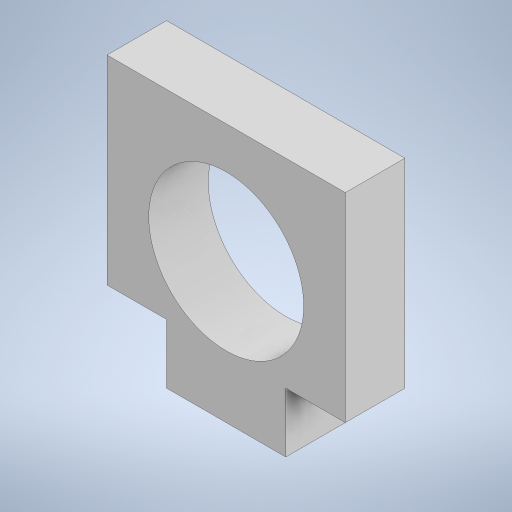
# Autodesk Inventor part: rod holder
Saved by Autodesk Inventor 2023 (Build 270158000, 158)
## iProperties
Created: 2023-11-14
Part Number: rod holder
Material: Generic
Document SubType Name: Modeling
Designer: Nate
Density: 1 g/cm^3
Appearance: Default
Author: Nate
Autodesk Inventor part; units mm, degrees
ref_plane "YZ Plane" through (0, 0, 0) normal (1, 0, 0) x (0, 1, 0)
ref_plane "XZ Plane" through (0, 0, 0) normal (0, 1, 0) x (-1, 0, 0)
ref_plane "XY Plane" through (0, 0, 0) normal (0, 0, 1) x (1, 0, 0)
sketch "Sketch1" plane through (0, 0, 0) normal (0, 0, 1) x (1, 0, 0)
  circle A0 centre (0, 0) radius 4.1275
  line L0 (-6.35, 6.35) -> (6.35, 6.35)
  line L1 (6.35, 6.35) -> (6.35, -4.2672)
  line L2 (6.35, -4.2672) -> (-6.35, -4.2672)
  line L3 (-6.35, -4.2672) -> (-6.35, 6.35)
  line L4 (-3.175, -4.2672) -> (3.175, -4.2672)
  line L5 (3.175, -4.2672) -> (3.175, -7.4422)
  line L6 (3.175, -7.4422) -> (-3.175, -7.4422)
  line L7 (-3.175, -7.4422) -> (-3.175, -4.2672)
  dimension "d0" = 8.255
  dimension "d1" = 4.2672
  dimension "d2" = 6.35
  dimension "d3" = 6.35
  dimension "d4" = 6.35
  dimension "d5" = 3.175
  dimension "d6" = 3.175
  dimension "d7" = 3.175
  constraints: 16 end point, 4 parallel, 2 horizontal, 2 perpendicular, 1 centre point, 1 coincident, 1 point on line
  measures "d0" diameter of A0
  measures "d1" distance from line of L2 A0.centre
  measures "d2" distance from line of A0.centre L1
  measures "d3" distance from line of L3 point (0, 0)
  measures "d4" distance from line of L0 A0.centre
  measures "d5" distance between parallel lines of L2 L6
  measures "d6" distance between parallel lines of L1 L5
  measures "d7" distance between parallel lines of L3 L7
extrude "Extrusion1" add sketch "Sketch1" along normal blind 3.175
body "Solid1"
